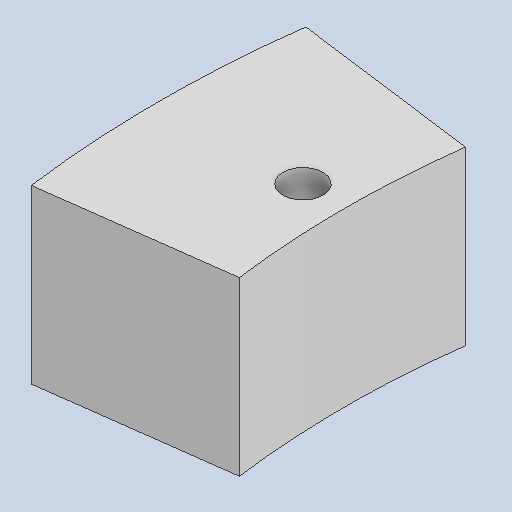
# Autodesk Inventor part: Spacer (make 5)
Saved by Autodesk Inventor 2025.1 (Build 291241020, 241B)
## iProperties
Created: 2024-12-11
Part Number: Spacer (make 5)
Material: Generic
Document SubType Name: Modeling
Designer: jdl5984
Density: 1 g/cm^3
Appearance: Default
Author: jdl5984
Autodesk Inventor part; units mm, degrees
ref_plane "YZ Plane" through (0, 0, 0) normal (1, 0, 0) x (0, 1, 0)
ref_plane "XZ Plane" through (0, 0, 0) normal (0, 1, 0) x (-1, 0, 0)
ref_plane "XY Plane" through (0, 0, 0) normal (0, 0, 1) x (1, 0, 0)
sketch "Sketch1" plane through (0, 0, 0) normal (0, 1, 0) x (-1, 0, 0)
  circle A0 centre (0, 0) radius 2.6543
  circle A1 centre (0, 0) radius 12.7 construction
  circle A2 centre (-120.65, 0) radius 120.65 construction
  arc A3 (5.2635, 16.5768) -> (5.2635, -16.5768) centre (-120.65, 0) ccw construction
  circle A4 centre (-120.65, 0) radius 92.075 construction
  line L0 (-120.65, 0) -> (17.8548, -18.2345)
  line L1 (-120.65, 0) -> (17.8548, 18.2345)
  line L2 (52.6661, 0) -> (-260.0292, 0) construction
  arc A5 (-6.5724, -15.0186) -> (-6.5724, 15.0186) centre (-120.65, 0) ccw
  circle A6 centre (-120.65, 0) radius 139.7
  point P0 (-5.588, 0)
  dimension "d4" = 241.3
  dimension "d0" = 5.3086
  dimension "d1" = 25.4
  dimension "d5" = 254
  dimension "d6" = 184.15
  dimension "d7" = 7.5
  dimension "d8" = 7.5
  dimension "d9" = 5.588
  dimension "d10" = 279.4
  constraints: 7 point on circle, 6 centre point, 6 coincident, 6 end point, 4 point on line, 1 horizontal, 1 horizontal alignment, 2 other
  measures "d0" diameter of A0
  measures "d1" diameter of A1
  measures "d5" diameter of A3
  measures "d6" diameter of A4
  measures "d7" angle of L0 L2
  measures "d8" angle of L1 L2
  measures "d9" distance of point (-5.588, 0) point (0, 0)
  measures "d10" diameter of A6
extrude "Extrusion1" add sketch "Sketch1" along normal blind 22.86 contours A5 L1 A6 L0
body "Solid1"
